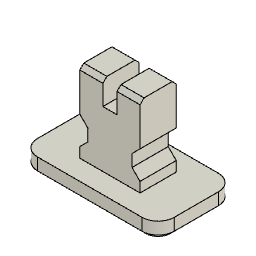
Switch_Slider_M1 (Autodesk Fusion 360 design; units mm, degrees)
Autodesk Fusion 360 part; units mm, degrees
note: some values were not read from the file. Set by a fixed rule: which sketch regions a step uses.
sketch "Skizze1" plane through (0, 0, 0) normal (0, 0, 1) x (1, 0, 0)
  line L0 (-6.5, 4.75) -> (6.5, 4.75)
  line L1 (8.5, 2.75) -> (8.5, -2.75)
  line L2 (6.5, -4.75) -> (-6.5, -4.75)
  line L3 (-8.5, -2.75) -> (-8.5, 2.75)
  line L4 (-8.5, 4.75) -> (8.5, -4.75) construction
  line L5 (8.5, 4.75) -> (-8.5, -4.75) construction
  arc A0 (8.5, 2.75) -> (6.5, 4.75) centre (6.5, 2.75) ccw
  arc A1 (-6.5, 4.75) -> (-8.5, 2.75) centre (-6.5, 2.75) ccw
  arc A2 (-8.5, -2.75) -> (-6.5, -4.75) centre (-6.5, -2.75) ccw
  arc A3 (6.5, -4.75) -> (8.5, -2.75) centre (6.5, -2.75) ccw
  dimension "d464" = 17
  dimension "d465" = 9.5
  dimension "d468" = 2
  constraint horizontal L0
  constraint perpendicular L0 L1
  constraint parallel L0 L2
  constraint parallel L1 L3
  constraint coincident L4 origin
  constraint coincident L5 origin
  constraint coincident L5.start L1
  constraint coincident L5.start L0
  constraint tangent L1 A0
  constraint tangent L0 A0
  constraint coincident L4.start L0
  constraint coincident L4.start L3
  constraint tangent L0 A1
  constraint tangent L3 A1
  constraint equal A0 A1
  constraint coincident L5.end L3
  constraint coincident L5.end L2
  constraint tangent L3 A2
  constraint tangent L2 A2
  constraint equal A0 A2
  constraint coincident L4.end L2
  constraint coincident L4.end L1
  constraint tangent L2 A3
  constraint tangent L1 A3
  constraint equal A0 A3
  measures "d464" distance of L4.end L5.end
  measures "d465" distance of L5.start L4.end
  measures "d468" radius of A0
extrude "Extrusion1" add sketch "Skizze1" along normal blind 2
sketch "Skizze2" plane through (0, 0, 2) normal (0, 0, 1) x (-1, 0, 0)
  arc A0 (8.5, 2.75) -> (6.5, 4.75) centre (6.5, 2.75) ccw
  line L0 (6.5, 4.75) -> (-6.5, 4.75)
  arc A1 (-6.5, 4.75) -> (-8.5, 2.75) centre (-6.5, 2.75) ccw
  line L1 (-8.5, 2.75) -> (-8.5, -2.75)
  arc A2 (-8.5, -2.75) -> (-6.5, -4.75) centre (-6.5, -2.75) ccw
  line L2 (-6.5, -4.75) -> (6.5, -4.75)
  arc A3 (6.5, -4.75) -> (8.5, -2.75) centre (6.5, -2.75) ccw
  line L3 (8.5, -2.75) -> (8.5, 2.75)
  line L4 (3.75, 2.25) -> (-3.75, 2.25)
  line L5 (-3.75, 2.25) -> (-3.75, -2.25)
  line L6 (-3.75, -2.25) -> (3.75, -2.25)
  line L7 (3.75, -2.25) -> (3.75, 2.25)
  line L8 (3.75, 2.25) -> (-3.75, -2.25) construction
  line L9 (-3.75, 2.25) -> (3.75, -2.25) construction
  dimension "d469" = 7.5
  dimension "d470" = 4.5
  constraint horizontal L4
  constraint perpendicular L4 L5
  constraint parallel L4 L6
  constraint parallel L5 L7
  constraint coincident L8 origin
  constraint coincident L9 origin
  measures "d469" distance of L5.end L6.end
  measures "d470" distance of L4.end L5.end
extrude "Extrusion2" add sketch "Skizze2" along normal blind 10 contours L4 L5 L6 L7
sketch "Skizze3" plane through (0, -2.25, 0) normal (0, -1, 0) x (1, 0, 0)
  line L0 (-3.75, 2) -> (3.75, 2)
  line L1 (3.75, 2) -> (3.75, 12)
  line L2 (3.75, 12) -> (-3.75, 12)
  line L3 (-3.75, 12) -> (-3.75, 2)
  line L4 (-0.875, 12) -> (0.875, 12)
  line L5 (0.875, 12) -> (0.875, 9)
  line L6 (0.875, 9) -> (-0.875, 9)
  line L7 (-0.875, 9) -> (-0.875, 12)
  line L8 (-0.875, 12) -> (0.875, 9) construction
  line L9 (0.875, 12) -> (-0.875, 9) construction
  line L10 (-3.75, 3.25) -> (-2.75, 4.25)
  line L11 (-3.75, 3.25) -> (-1.5, 3.25) construction
  line L12 (-2.75, 4.25) -> (-2.75, 5.75)
  line L13 (-2.75, 5.75) -> (-3.75, 6.75)
  line L14 (-6.5, 2) -> (6.5, 2)
  line L15 (0, 20) -> (0, 2.5)
  line L16 (3.75, 3.25) -> (2.75, 4.25)
  line L17 (2.75, 4.25) -> (2.75, 5.75)
  line L18 (2.75, 5.75) -> (3.75, 6.75)
  point P0 (0, 10.5)
  dimension "d479" = 1.75
  dimension "d480" = 3
  dimension "d483" = 45
  dimension "d484" = 1
  dimension "d485" = 1.5
  dimension "d486" = 2.25
  constraint horizontal L4
  constraint perpendicular L4 L5
  constraint parallel L4 L6
  constraint parallel L5 L7
  constraint coincident L8 P0
  constraint coincident L9 P0
  constraint vertical origin P0
  constraint coincident L2 L4.start
  constraint horizontal L11
  constraint coincident L3 L10.start
  constraint parallel L3 L12
  constraint coincident L3 L13.end
  constraint equal L10 L13
  constraint symmetric L10.start L15 L16.start
  constraint symmetric L10.end L15 L16.end
  constraint symmetric L12.end L15 L17.end
  constraint symmetric L13.end L15 L18.end
  measures "d479" distance of L4.start L4.end
  measures "d480" distance of L4.end L5.end
  measures "d483" angle of L10 L11
  measures "d484" distance of L3 L12
  measures "d485" distance of L10.end L12.end
  measures "d486" distance of L10.end L14
extrude "Extrusion3" cut sketch "Skizze3" against normal up to surface (4.5 mm away) contours L3 L10 L12 L13 | L1 L16 L17 L18 | L2 L4 L6 L7 L15 | L2 L4 L5 L6 L15
sketch "Skizze4" plane through (0, 0, 0) normal (0, 0, -1) x (1, 0, 0)
  arc A0 (-6.5, 4.75) -> (-8.5, 2.75) centre (-6.5, 2.75) ccw
  line L0 (-8.5, 2.75) -> (-8.5, -2.75)
  arc A1 (-8.5, -2.75) -> (-6.5, -4.75) centre (-6.5, -2.75) ccw
  line L1 (-6.5, -4.75) -> (6.5, -4.75)
  arc A2 (6.5, -4.75) -> (8.5, -2.75) centre (6.5, -2.75) ccw
  line L2 (8.5, -2.75) -> (8.5, 2.75)
  arc A3 (8.5, 2.75) -> (6.5, 4.75) centre (6.5, 2.75) ccw
  line L3 (6.5, 4.75) -> (-6.5, 4.75)
  line L4 (-1, 3.5) -> (1, 3.5)
  line L5 (1, 3.5) -> (1, -3.5)
  line L6 (1, -3.5) -> (-1, -3.5)
  line L7 (-1, -3.5) -> (-1, 3.5)
  line L8 (-1, 3.5) -> (1, -3.5) construction
  line L9 (1, 3.5) -> (-1, -3.5) construction
  line L10 (-5.5, 3.5) -> (-3.5, 3.5)
  line L11 (-3.5, 3.5) -> (-3.5, -3.5)
  line L12 (-3.5, -3.5) -> (-5.5, -3.5)
  line L13 (-5.5, -3.5) -> (-5.5, 3.5)
  line L14 (-5.5, 3.5) -> (-3.5, -3.5) construction
  line L15 (-3.5, 3.5) -> (-5.5, -3.5) construction
  line L16 (3.5, 3.5) -> (5.5, 3.5)
  line L17 (5.5, 3.5) -> (5.5, -3.5)
  line L18 (5.5, -3.5) -> (3.5, -3.5)
  line L19 (3.5, -3.5) -> (3.5, 3.5)
  line L20 (3.5, 3.5) -> (5.5, -3.5) construction
  line L21 (5.5, 3.5) -> (3.5, -3.5) construction
  point P0 (-4.5, 0)
  point P1 (4.5, 0)
  dimension "d503" = 2
  dimension "d504" = 7
  dimension "d505" = 2.5
  dimension "d506" = 2.5
  constraint horizontal L4
  constraint perpendicular L4 L5
  constraint parallel L4 L6
  constraint parallel L5 L7
  constraint coincident L8 origin
  constraint coincident L9 origin
  constraint horizontal L10
  constraint perpendicular L10 L11
  constraint parallel L10 L12
  constraint parallel L11 L13
  constraint coincident L14 P0
  constraint coincident L15 P0
  constraint horizontal L16
  constraint perpendicular L16 L17
  constraint parallel L16 L18
  constraint parallel L17 L19
  constraint coincident L20 P1
  constraint coincident L21 P1
  constraint horizontal origin P1
  constraint horizontal origin P0
  constraint equal L6 L18
  constraint equal L6 L12
  constraint horizontal L6.end L11.end
  constraint horizontal L5.end L18.end
  measures "d503" distance of L5.end L6.end
  measures "d504" distance of L4.end L5.end
  measures "d505" distance of L4.end L16.start
  measures "d506" distance of L4.start L10.end
extrude "Extrusion4" cut sketch "Skizze4" against normal blind 0.5 contours L4 L5 L6 L7 | L10 L11 L12 L13 | L16 L17 L18 L19
chamfer "Fase1" distance 0.5 angle 45 12 edges at (-7.9142, -4.1642, 0) (0, -4.75, 0) (7.9142, -4.1642, 0) (8.5, 0, 0) (7.9142, 4.1642, 0) (0, 4.75, 0) (-7.9142, 4.1642, 0) (-8.5, 0, 0) (-2.3125, -2.25, 12) (2.3125, -2.25, 12) (-2.3125, 2.25, 12) (2.3125, 2.25, 12)
equation "d465 = 10 mm - ( 2 * 0.25 ) * 1 mm"
equation "d469 = 10 mm - 2.5 mm"
equation "d470 = 5 mm - ( 2 * 0.25 ) * 1 mm"
equation "d486 = 2 mm + 0.25 mm"
equation "d506 = d505"
